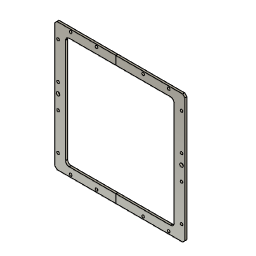
1006350A-3dprint-GASKET, RETAINED (Autodesk Fusion 360 design; units mm, degrees)
Autodesk Fusion 360 part; units mm, degrees
note: some values were not read from the file. Set by a fixed rule: the direction of a hole.
sketch "Front" plane through (0, 0, 0) normal (0, 1, 0) x (1, 0, 0) in component "1006350A"
  line L0 (-97.5923, -201.9946) -> (221.2351, -201.9946) construction
  line L1 (-99.947, -6.4146) -> (290.3014, -6.4146) construction
  line L2 (12.4997, 61.7326) -> (12.4997, -271.4585) construction
  line L3 (208.0797, 69.9741) -> (208.0797, -187.16) construction
  line L4 (213.4645, 13.4611) -> (213.4645, -265.3363) construction
  line L5 (7.1149, -256.6239) -> (7.1149, 6.397) construction
  line L6 (-10.9391, -2.6046) -> (257.2621, -2.6046) construction
  line L7 (3.4246, -205.8046) -> (275.1579, -205.8046) construction
  line L8 (196.1925, -231.664) -> (196.1925, 4.0423) construction
  line L9 (200.5105, 72.0933) -> (200.5105, -273.8132) construction
  line L10 (20.3229, -271.4585) -> (20.3229, 19.5833) construction
  line L11 (-9.5263, -26.3536) -> (218.174, -26.3536) construction
  line L12 (-30.2477, -84.6466) -> (216.2902, -84.6466) construction
  line L13 (226.8864, -107.3796) -> (-21.2998, -107.3796) construction
  line L14 (-47.6725, -123.7626) -> (220.7641, -123.7626) construction
  line L15 (-72.1615, -182.0556) -> (219.1158, -182.0556) construction
  line L16 (-7.1716, -192.3426) -> (237.718, -192.3426) construction
  line L17 (24.3869, -243.673) -> (24.3869, 8.2807) construction
  line L18 (187.7982, 11.5773) -> (187.7982, -213.2972) construction
  line L19 (147.2467, 23.5863) -> (147.2467, -210.9425) construction
  line L20 (73.3327, 36.3018) -> (73.3327, -224.8353) construction
  line L21 (32.4133, 51.8428) -> (32.4133, -217.3002) construction
  line L22 (267.4197, -11.8756) -> (2.5805, -11.8756) construction
  line L23 (267.0325, -196.4066) -> (1.4189, -196.4066) construction
  line L24 (1.5972, -16.0666) -> (220.1148, -16.0666) construction
  line L25 (7.1149, -205.8046) -> (213.4645, -205.8046)
  line L26 (213.4645, -205.8046) -> (213.4645, -2.6046)
  line L27 (213.4645, -2.6046) -> (7.1149, -2.6046)
  line L28 (7.1149, -2.6046) -> (7.1149, -205.8046)
  line L29 (24.3869, -192.3426) -> (196.1925, -192.3426)
  line L30 (196.1925, -192.3426) -> (196.1925, -16.0666)
  line L31 (196.1925, -16.0666) -> (24.3869, -16.0666)
  line L32 (24.3869, -16.0666) -> (24.3869, -192.3426)
  point P0 (32.4133, -201.9946)
  point P1 (73.3327, -201.9946)
  point P2 (147.2467, -201.9946)
  point P3 (187.7982, -201.9946)
  point P4 (208.0797, -182.0556)
  point P5 (208.0797, -123.7626)
  point P6 (208.0797, -107.3796)
  point P7 (208.0797, -84.6466)
  point P8 (208.0797, -26.3536)
  point P9 (187.7982, -6.4146)
  point P10 (147.2467, -6.4146)
  point P11 (73.3327, -6.4146)
  point P12 (32.4133, -6.4146)
  point P13 (12.4997, -26.3536)
  point P14 (12.4997, -84.6466)
  point P15 (12.4997, -107.3796)
  point P16 (12.4997, -123.7626)
  point P17 (12.4997, -182.0556)
  dimension "d1" = 195.58
  dimension "d2" = 3.81
  dimension "d3" = 19.939
  dimension "d4" = 78.232
  dimension "d5" = 117.348
  dimension "d6" = 175.641
  dimension "d7" = 100.965
  dimension "d10" = 5.3848
  dimension "d11" = 17.272
  dimension "d12" = 60.833
  dimension "d13" = 134.747
  dimension "d14" = 175.6664
  dimension "d15" = 195.58
  dimension "d16" = 203.2
  dimension "d17" = 184.531
  dimension "d18" = 5.461
  dimension "d19" = 13.462
  dimension "d20" = 189.0776
  dimension "d21" = 206.3496
  dimension "d22" = 13.462
  dimension "d33" = 7.5692
  dimension "d34" = 180.1876
  constraint horizontal L0
  constraint horizontal L1
  constraint perpendicular L0 L2
  constraint perpendicular L0 L3
  constraint parallel L3 L4
  constraint parallel L2 L5
  constraint perpendicular L2 L6
  constraint perpendicular L4 L7
  constraint perpendicular L6 L8
  constraint perpendicular L7 L9
  constraint perpendicular L6 L10
  constraint perpendicular L4 L11
  constraint perpendicular L4 L12
  constraint perpendicular L4 L13
  constraint perpendicular L8 L14
  constraint perpendicular L4 L15
  constraint perpendicular L4 L16
  constraint perpendicular L6 L17
  constraint perpendicular L7 L18
  constraint perpendicular L7 L19
  constraint perpendicular L6 L20
  constraint perpendicular L7 L21
  constraint perpendicular L5 L22
  constraint perpendicular L5 L23
  constraint perpendicular L4 L24
  constraint coincident L5 L25.start
  constraint coincident L7 L25.start
  constraint coincident L4 L25.end
  constraint coincident L7 L25.end
  constraint coincident L4 L26.end
  constraint coincident L6 L26.end
  constraint coincident L5 L27.end
  constraint coincident L6 L27.end
  constraint coincident L17 L29.start
  constraint coincident L16 L29.start
  constraint coincident L8 L29.end
  constraint coincident L16 L29.end
  constraint coincident L8 L30.end
  constraint coincident L24 L30.end
  constraint coincident L24 L31.end
  constraint coincident L17 L31.end
  constraint coincident L21 P0
  constraint coincident L0 P0
  constraint coincident L0 P1
  constraint coincident L20 P1
  constraint coincident L0 P2
  constraint coincident L19 P2
  constraint coincident L18 P3
  constraint coincident L0 P3
  constraint coincident L15 P4
  constraint coincident L3 P4
  constraint coincident L3 P5
  constraint coincident L14 P5
  constraint coincident L3 P6
  constraint coincident L13 P6
  constraint coincident L3 P7
  constraint coincident L12 P7
  constraint coincident L11 P8
  constraint coincident L3 P8
  constraint coincident L1 P9
  constraint coincident L18 P9
  constraint coincident L1 P10
  constraint coincident L19 P10
  constraint coincident L20 P11
  constraint coincident L1 P11
  constraint coincident L1 P12
  constraint coincident L21 P12
  constraint coincident L2 P13
  constraint coincident L11 P13
  constraint coincident L12 P14
  constraint coincident L2 P14
  constraint coincident L13 P15
  constraint coincident L2 P15
  constraint coincident L2 P16
  constraint coincident L14 P16
  constraint coincident L15 P17
  constraint coincident L2 P17
  measures "d1" distance of L0 L1
  measures "d2" distance of L1 L6
  measures "d3" distance of L1 L11
  measures "d4" distance of L1 L12
  measures "d5" distance of L1 L14
  measures "d6" distance of L1 L15
  measures "d7" distance of L1 L13
  measures "d10" distance of L3 L4
  measures "d11" distance of L4 L8
  measures "d12" distance of L3 L19
  measures "d13" distance of L3 L20
  measures "d14" distance of L3 L21
  measures "d15" distance of L2 L3
  measures "d16" distance of L6 L7
  measures "d17" distance of L22 L23
  measures "d18" distance of L1 L22
  measures "d19" distance of L6 L24
  measures "d20" distance of L4 L17
  measures "d21" distance of L4 L5
  measures "d22" distance of L7 L16
  measures "d33" distance of L3 L9
  measures "d34" distance of L9 L10
extrude "Extrude1" add sketch "Front" along normal blind 3.175 makes body 1 in component "1006350A"
chamfer "Chamfer1" distance 3.556 angle 45 4 edges at (7.1149, 1.5875, 205.8046) (213.4645, 1.5875, 205.8046) (213.4645, 1.5875, 2.6046) (7.1149, 1.5875, 2.6046) on bodies 1 in component "1006350A"
fillet "Fillet1" radius 5.5372 4 edges at (196.1925, 1.5875, 192.3426) (24.3869, 1.5875, 192.3426) (24.3869, 1.5875, 16.0666) (196.1925, 1.5875, 16.0666) on bodies 1 in component "1006350A"
hole "Hole1" at (12.4997, 0, 107.3796) at (208.0797, 0, 107.3796) direction (0, 1, 0) diameter 5.5372 end through all bodies 1 in component "1006350A"
hole "Hole2" at (147.2467, 0, 201.9946) at (187.7982, 0, 201.9946) at (208.0797, 0, 182.0556) at (208.0797, 0, 123.7626) at (73.3327, 0, 201.9946) at (32.4133, 0, 201.9946) at (12.4997, 0, 182.0556) at (12.4997, 0, 123.7626) at (12.4997, 0, 84.6466) at (12.4997, 0, 26.3536) at (32.4133, 0, 6.4146) at (73.3327, 0, 6.4146) at (147.2467, 0, 6.4146) at (187.7982, 0, 6.4146) at (208.0797, 0, 26.3536) at (208.0797, 0, 84.6466) direction (0, 1, 0) diameter 4.0894 end through all bodies 1 in component "1006350A"
ref_plane "WorkPlane1" through (104.14, 0, 0) normal (1, 0, 0) x (0, 1, 0)
split "Split1" by plane through (104.14, 0, 0) normal (1, 0, 0) bodies 1 makes body 2 at (117.8444, 0, 199.8956) in component "1006350A"
component "1006350A" placed x (1, 0, 0) y (0, 1, 0) z (0, 0, 1) at (0, 0, 0)
named bodies: "1006350A-Left-half", "1006350A-Right-half"
